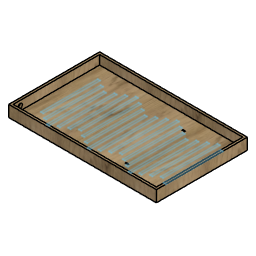
Dissertation_demo v1 v0 (Autodesk Fusion 360 design; units mm, degrees)
Autodesk Fusion 360 part; units mm, degrees
sketch "Sketch1" plane through (0, 0, 0) normal (0, 0, 1) x (1, 0, 0) in component "Component'"
  line L0 (211.4953, 133.158) -> (206.4953, 133.158)
  line L1 (206.4953, 133.158) -> (206.4953, 127.158)
  line L2 (206.4953, 127.158) -> (211.4953, 127.158)
  line L3 (211.4953, 127.158) -> (211.4953, 133.158)
  dimension "d10" = 5
  dimension "d11" = 6
  constraint horizontal L0
  constraint vertical L1
  constraint horizontal L2
  constraint vertical L3
  measures "d10" distance of L0.start L0.end
  measures "d11" distance of L0.start L2.end
extrude "Extrude1" add sketch "Sketch1" against normal blind 3 makes body 1 in component "Component'"
copy_body "CopyPasteBodies1" bodies 1 makes body 2 in component "Component'"
move_body "Move1" bodies 2 to x (1, 0, 0) y (0, 1, 0) z (0, 0, 1) at (0, -17, 0) in component "Component'"
copy_body "CopyPasteBodies2" bodies 1 2 makes body 3 makes body 4 in component "Component'"
move_body "Move2" bodies 3 4 to x (1, 0, 0) y (0, 1, 0) z (0, 0, 1) at (0, -35, 0) in component "Component'"
copy_body "CopyPasteBodies3" bodies 1 2 3 4 makes body 5 makes body 6 makes body 7 makes body 8 in component "Component'"
move_body "Move3" bodies 5 6 7 8 to x (1, 0, 0) y (0, 1, 0) z (0, 0, 1) at (0, -68, 0) in component "Component'"
copy_body "CopyPasteBodies4" bodies 1 2 3 4 5 6 7 makes body 9 makes body 10 makes body 11 makes body 12 makes body 13 makes body 14 makes body 15 in component "Component'"
move_body "Move4" bodies 9 10 11 12 13 14 15 to x (1, 0, 0) y (0, 1, 0) z (0, 0, 1) at (0, -136, 0) in component "Component'"
sketch "Sketch2" plane through (0, 0, 0) normal (0, 0, 1) x (1, 0, 0) in component "Component'"
  line L0 (213.9024, 135.458) -> (203.9024, 135.458)
  line L1 (203.9024, 135.458) -> (203.9024, -114.542)
  line L2 (203.9024, -114.542) -> (213.9024, -114.542)
  line L3 (213.9024, -114.542) -> (213.9024, 135.458)
  dimension "d14" = 10
  dimension "d15" = 250
  constraint horizontal L0
  constraint vertical L1
  constraint horizontal L2
  constraint vertical L3
  measures "d14" distance of L0.start L0.end
  measures "d15" distance of L0.start L2.end
extrude "Extrude2" cut sketch "Sketch2" against normal blind 1 bodies 1 2 3 4 5 6 7 8 9 10 11 12 13 14 15 in component "Component'"
move_body "Move5" bodies 1 2 3 4 5 6 7 9 8 10 12 13 14 15 11 to x (1, 0, 0) y (0, 1, 0) z (0, 0, 1) at (0, 0, -1) in component "Component'"
extrude "Extrude4" add sketch "Sketch2" against normal blind 1 separate body makes body 16 in component "Component'"
sketch "Sketch1 (2)" plane through (0, 0, 0) normal (0, 0, 1) x (1, 0, 0) in component "Main"
  line L0 (-250, 200) -> (250, 200)
  line L1 (250, 200) -> (250, -200)
  line L2 (250, -200) -> (-250, -200)
  line L3 (-250, -200) -> (-250, 200)
  line L4 (-250, 200) -> (250, -200) construction
  line L5 (250, 200) -> (-250, -200) construction
  line L6 (-240, 190) -> (240, 190)
  line L7 (240, 190) -> (240, -190)
  line L8 (240, -190) -> (-240, -190)
  line L9 (-240, -190) -> (-240, 190)
  dimension "d26" = 500
  dimension "d27" = 400
  dimension "d28" = 10
  constraint horizontal L0
  constraint perpendicular L0 L1
  constraint parallel L0 L2
  constraint parallel L1 L3
  constraint coincident L4 origin
  constraint coincident L5 origin
  measures "d26" distance of L1.end L2.end
  measures "d27" distance of L0.end L1.end
extrude "Extrude1'" add sketch "Sketch1 (2)" along normal blind 50 separate body makes body 17 in component "Main"
extrude "Extrude3" add sketch "Sketch1 (2)" along normal blind 10 contours L6 L7 L8 L9 bodies 17 in component "Main"
sketch "Sketch2 (2)" plane through (0, 0, 0) normal (0, 0, 1) x (1, 0, 0) in component "Main"
sketch "Sketch3" plane through (0, 0, 0) normal (0, 0, 1) x (1, 0, 0) in component "Main"
  line L0 (201, 127) -> (189, 127)
  line L1 (189, 127) -> (189, 123)
  line L2 (189, 123) -> (201, 123)
  line L3 (201, 123) -> (201, 127)
  dimension "d35" = 12
  dimension "d36" = 4
  constraint horizontal L0
  constraint vertical L1
  constraint horizontal L2
  constraint vertical L3
  measures "d35" distance of L0.start L0.end
  measures "d36" distance of L0.start L2.end
extrude "Extrude4'" cut sketch "Sketch3" along normal blind 10 bodies 17 in component "Main"
sketch "Sketch4" plane through (-13.9, -10.5, 0) normal (0, 0, 1) x (1, 0, 0) in component "Main"
  line L0 (214.9, -116.5) -> (202.9, -116.5)
  line L1 (202.9, -116.5) -> (202.9, -112.5)
  line L2 (202.9, -112.5) -> (214.9, -112.5)
  line L3 (214.9, -112.5) -> (214.9, -116.5)
  dimension "d39" = 12
  dimension "d40" = 4
  constraint horizontal L0
  constraint vertical L1
  constraint horizontal L2
  constraint vertical L3
  measures "d39" distance of L0.start L0.end
  measures "d40" distance of L0.start L2.end
extrude "Extrude5" cut sketch "Sketch4" along normal blind 10 bodies 17 in component "Main"
sketch "Sketch1 (3)" plane through (0, 0, 0) normal (0, 0, 1) x (1, 0, 0) in component "Component''"
  line L0 (202.6, 125) -> (187.4, 125)
  line L1 (187.4, 125) -> (187.4, -125)
  line L2 (187.4, -125) -> (202.6, -125)
  line L3 (202.6, -125) -> (202.6, 125)
  dimension "d43" = 15.2
  dimension "d44" = 250
  constraint horizontal L0
  constraint vertical L1
  constraint horizontal L2
  constraint vertical L3
  measures "d43" distance of L0.start L0.end
  measures "d44" distance of L0.start L2.end
extrude "Extrude1''" add sketch "Sketch1 (3)" against normal blind 5 separate body makes body 18 in component "Component''"
sketch "Sketch2 (3)" plane through (0, -125, 0) normal (0, -1, 0) x (1, 0, 0) in component "Component''"
  line L0 (202.6, 0) -> (187.4, 0)
  line L1 (187.4, 0) -> (187.4, -5)
  line L2 (187.4, -5) -> (202.6, -5)
  line L3 (202.6, -5) -> (202.6, 0)
  line L4 (202, 0) -> (188, 0)
  line L5 (188, 0) -> (188, -4)
  line L6 (188, -4) -> (202, -4)
  line L7 (202, -4) -> (202, 0)
  constraint horizontal L4
  constraint vertical L5
  constraint horizontal L6
  constraint vertical L7
  constraint coincident L0 L4.start
extrude "Extrude2'" cut sketch "Sketch2 (3)" against normal blind 250 contours L0 L4 L5 L6 L7 bodies 18 in component "Component''"
hole "Hole1" at (-250, -159.5585, 28.611) direction (1, 0, 0) diameter 20 depth 110 tip angle 118 bodies 17 in component "Main"
move_face "OffsetFaces1" offset 150 1 faces at (250, 66.6667, 33.3333) on bodies 17 in component "Main"
sketch "Sketch1 (4)" plane through (0, 0, 50) normal (0, 0, 1) x (-1, 0, 0)
  line L0 (-240, 190) -> (240, 190)
  line L1 (240, 190) -> (240, -190)
  line L2 (240, -190) -> (-240, -190)
  line L3 (-240, -190) -> (-240, 190)
  line L4 (250, 200) -> (-400, 200)
  line L5 (-400, 200) -> (-400, -200)
  line L6 (-400, -200) -> (250, -200)
  line L7 (250, -200) -> (250, 200)
  line L8 (-240, 190) -> (-390, 190)
  line L9 (-390, 190) -> (-390, -190)
  line L10 (-390, -190) -> (-240, -190)
  line L11 (-240, -190) -> (-240, 190)
  constraint horizontal L8
  constraint vertical L9
  constraint horizontal L10
  constraint vertical L11
  constraint coincident L0.start L3.end
extrude "Extrude6" cut sketch "Sketch1 (4)" against normal blind 40 contours L3 L8 L9 L10 L11 bodies 17 in component "Main"
sketch "Sketch2 (4)" plane through (0, 0, 0) normal (0, 0, -1) x (1, 0, 0)
  line L0 (201, 127) -> (201, 123)
  line L1 (201, 123) -> (189, 123)
  line L2 (189, 123) -> (189, 127)
  line L3 (189, 127) -> (201, 127)
  line L4 (189, -123) -> (201, -123)
  line L5 (201, -123) -> (201, -127)
  line L6 (201, -127) -> (189, -127)
  line L7 (189, -127) -> (189, -123)
  line L8 (400, 200) -> (-250, 200)
  line L9 (-250, 200) -> (-250, -200)
  line L10 (-250, -200) -> (400, -200)
  line L11 (400, -200) -> (400, 200)
  line L12 (374.7896, 142.4931) -> (372.7896, 142.4931)
  line L13 (372.7896, 142.4931) -> (372.7896, 162.4931)
  line L14 (372.7896, 162.4931) -> (374.7896, 162.4931)
  line L15 (374.7896, 162.4931) -> (374.7896, 142.4931)
  line L16 (352.7896, 162.4931) -> (352.7896, 142.4931)
  line L17 (352.7896, 142.4931) -> (350.7896, 142.4931)
  line L18 (350.7896, 142.4931) -> (350.7896, 162.4931)
  line L19 (350.7896, 162.4931) -> (352.7896, 162.4931)
  dimension "d55" = 2
  dimension "d56" = 20
  dimension "d59" = -22
  dimension "d60" = 0
  constraint horizontal L12
  constraint vertical L13
  constraint horizontal L14
  constraint vertical L15
  measures "d55" distance of L12.start L12.end
  measures "d56" distance of L12.start L14.end
extrude "Extrude7" cut sketch "Sketch2 (4)" against normal blind 49 contours L12 L13 L14 L15 | L16 L17 L18 L19 bodies 17 in component "Main"
sketch "Sketch3 (2)" plane through (0, 0, 0) normal (0, 0, -1) x (1, 0, 0)
  line L0 (372.7896, 142.4931) -> (372.7896, 162.4931)
  line L1 (372.7896, 162.4931) -> (374.7896, 162.4931)
  line L2 (374.7896, 162.4931) -> (374.7896, 142.4931)
  line L3 (374.7896, 142.4931) -> (372.7896, 142.4931)
  line L4 (352.7896, 142.4931) -> (350.7896, 142.4931)
  line L5 (350.7896, 142.4931) -> (350.7896, 162.4931)
  line L6 (350.7896, 162.4931) -> (352.7896, 162.4931)
  line L7 (352.7896, 162.4931) -> (352.7896, 142.4931)
  line L8 (201, 127) -> (201, 123)
  line L9 (201, 123) -> (189, 123)
  line L10 (189, 123) -> (189, 127)
  line L11 (189, 127) -> (201, 127)
  line L12 (189, -123) -> (201, -123)
  line L13 (201, -123) -> (201, -127)
  line L14 (201, -127) -> (189, -127)
  line L15 (189, -127) -> (189, -123)
  line L16 (400, 200) -> (-250, 200)
  line L17 (-250, 200) -> (-250, -200)
  line L18 (-250, -200) -> (400, -200)
  line L19 (400, -200) -> (400, 200)
  line L20 (370.7864, 140.5007) -> (368.7864, 140.5007)
  line L21 (368.7864, 140.5007) -> (368.7864, 164.5007)
  line L22 (368.7864, 164.5007) -> (370.7864, 164.5007)
  line L23 (370.7864, 164.5007) -> (370.7864, 140.5007)
  line L24 (356.7864, 140.5007) -> (354.7864, 140.5007)
  line L25 (356.7864, 164.5007) -> (356.7864, 140.5007)
  line L26 (354.7864, 140.5007) -> (354.7864, 164.5007)
  line L27 (354.7864, 164.5007) -> (356.7864, 164.5007)
  dimension "d63" = 2
  dimension "d64" = 24
  dimension "d67" = -14
  dimension "d68" = 0
  constraint horizontal L20
  constraint vertical L21
  constraint horizontal L22
  constraint vertical L23
  measures "d63" distance of L20.start L20.end
  measures "d64" distance of L20.start L22.end
extrude "Extrude8" cut sketch "Sketch3 (2)" against normal blind 12 contours L20 L21 L22 L23 | L24 L25 L26 L27 bodies 17 in component "Main"
sketch "Sketch4 (2)" plane through (0, 0, 0) normal (0, 0, -1) x (1, 0, 0)
  line L0 (368.7864, 140.5007) -> (368.7864, 164.5007)
  line L1 (368.7864, 164.5007) -> (370.7864, 164.5007)
  line L2 (370.7864, 164.5007) -> (370.7864, 140.5007)
  line L3 (370.7864, 140.5007) -> (368.7864, 140.5007)
  line L4 (356.7864, 140.5007) -> (354.7864, 140.5007)
  line L5 (354.7864, 140.5007) -> (354.7864, 164.5007)
  line L6 (354.7864, 164.5007) -> (356.7864, 164.5007)
  line L7 (356.7864, 164.5007) -> (356.7864, 140.5007)
  line L8 (372.7896, 142.4931) -> (372.7896, 162.4931)
  line L9 (372.7896, 162.4931) -> (374.7896, 162.4931)
  line L10 (374.7896, 162.4931) -> (374.7896, 142.4931)
  line L11 (374.7896, 142.4931) -> (372.7896, 142.4931)
  line L12 (352.7896, 142.4931) -> (350.7896, 142.4931)
  line L13 (350.7896, 142.4931) -> (350.7896, 162.4931)
  line L14 (350.7896, 162.4931) -> (352.7896, 162.4931)
  line L15 (352.7896, 162.4931) -> (352.7896, 142.4931)
  line L16 (201, 127) -> (201, 123)
  line L17 (201, 123) -> (189, 123)
  line L18 (189, 123) -> (189, 127)
  line L19 (189, 127) -> (201, 127)
  line L20 (189, -123) -> (201, -123)
  line L21 (201, -123) -> (201, -127)
  line L22 (201, -127) -> (189, -127)
  line L23 (189, -127) -> (189, -123)
  line L24 (400, 200) -> (-250, 200)
  line L25 (-250, 200) -> (-250, -200)
  line L26 (-250, -200) -> (400, -200)
  line L27 (400, -200) -> (400, 200)
  line L28 (366.8, 138.5) -> (364.8, 138.5)
  line L29 (364.8, 138.5) -> (364.8, 166.5)
  line L30 (364.8, 166.5) -> (366.8, 166.5)
  line L31 (366.8, 166.5) -> (366.8, 138.5)
  line L32 (360.8, 166.5) -> (360.8, 138.5)
  line L33 (360.8, 138.5) -> (358.8, 138.5)
  line L34 (358.8, 138.5) -> (358.8, 166.5)
  line L35 (358.8, 166.5) -> (360.8, 166.5)
  dimension "d73" = 2
  dimension "d74" = 28
  dimension "d77" = -6
  dimension "d78" = 0
  constraint horizontal L28
  constraint vertical L29
  constraint horizontal L30
  constraint vertical L31
  measures "d73" distance of L28.start L28.end
  measures "d74" distance of L28.start L30.end
sketch "Sketch5" plane through (0, 0, 0) normal (0, 0, -1) x (1, 0, 0)
  line L0 (367.5861, 138.8564) -> (365.5861, 138.8564)
  line L1 (365.5861, 138.8564) -> (365.5861, 166.8564)
  line L2 (365.5861, 166.8564) -> (367.5861, 166.8564)
  line L3 (367.5861, 166.8564) -> (367.5861, 138.8564)
  dimension "d71" = 2
  dimension "d72" = 28
  constraint horizontal L0
  constraint vertical L1
  constraint horizontal L2
  constraint vertical L3
  measures "d71" distance of L0.start L0.end
  measures "d72" distance of L0.start L2.end
extrude "Extrude9" cut sketch "Sketch4 (2)" against normal blind 10 contours L28 L29 L30 L31 | L32 L33 L34 L35 bodies 17 in component "Main"
sketch "Sketch6" plane through (0, 0, 0) normal (0, 0, -1) x (1, 0, 0)
  line L0 (364.8, 138.5) -> (364.8, 166.5)
  line L1 (364.8, 166.5) -> (366.8, 166.5)
  line L2 (366.8, 166.5) -> (366.8, 138.5)
  line L3 (366.8, 138.5) -> (364.8, 138.5)
  line L4 (360.8, 138.5) -> (358.8, 138.5)
  line L5 (358.8, 138.5) -> (358.8, 166.5)
  line L6 (358.8, 166.5) -> (360.8, 166.5)
  line L7 (360.8, 166.5) -> (360.8, 138.5)
  line L8 (368.7864, 140.5007) -> (368.7864, 164.5007)
  line L9 (368.7864, 164.5007) -> (370.7864, 164.5007)
  line L10 (370.7864, 164.5007) -> (370.7864, 140.5007)
  line L11 (370.7864, 140.5007) -> (368.7864, 140.5007)
  line L12 (356.7864, 140.5007) -> (354.7864, 140.5007)
  line L13 (354.7864, 140.5007) -> (354.7864, 164.5007)
  line L14 (354.7864, 164.5007) -> (356.7864, 164.5007)
  line L15 (356.7864, 164.5007) -> (356.7864, 140.5007)
  line L16 (372.7896, 142.4931) -> (372.7896, 162.4931)
  line L17 (372.7896, 162.4931) -> (374.7896, 162.4931)
  line L18 (374.7896, 162.4931) -> (374.7896, 142.4931)
  line L19 (374.7896, 142.4931) -> (372.7896, 142.4931)
  line L20 (352.7896, 142.4931) -> (350.7896, 142.4931)
  line L21 (350.7896, 142.4931) -> (350.7896, 162.4931)
  line L22 (350.7896, 162.4931) -> (352.7896, 162.4931)
  line L23 (352.7896, 162.4931) -> (352.7896, 142.4931)
  line L24 (201, 127) -> (201, 123)
  line L25 (201, 123) -> (189, 123)
  line L26 (189, 123) -> (189, 127)
  line L27 (189, 127) -> (201, 127)
  line L28 (189, -123) -> (201, -123)
  line L29 (201, -123) -> (201, -127)
  line L30 (201, -127) -> (189, -127)
  line L31 (189, -127) -> (189, -123)
  line L32 (400, 200) -> (-250, 200)
  line L33 (-250, 200) -> (-250, -200)
  line L34 (-250, -200) -> (400, -200)
  line L35 (400, -200) -> (400, 200)
  line L36 (363.7997, 136.5) -> (361.7997, 136.5)
  line L37 (361.7997, 136.5) -> (361.7997, 168.5)
  line L38 (361.7997, 168.5) -> (363.7997, 168.5)
  line L39 (363.7997, 168.5) -> (363.7997, 136.5)
  dimension "d81" = 2
  dimension "d82" = 32
  constraint horizontal L36
  constraint vertical L37
  constraint horizontal L38
  constraint vertical L39
  measures "d81" distance of L36.start L36.end
  measures "d82" distance of L36.start L38.end
extrude "Extrude10" cut sketch "Sketch6" against normal blind 31 contours L36 L37 L38 L39 bodies 17 in component "Main"
extrude "Extrude2''" [suppressed] in component "Main"
extrude "Extrude3'" [suppressed] in component "Component'"
sketch "Sketch1 (5)" plane through (0, 0, 0) normal (0, 0, -1) x (1, 0, 0) in component "Component"
  line L0 (140, 190) -> (-140, 190)
  line L1 (-140, 190) -> (-140, -190)
  line L2 (-140, -190) -> (140, -190)
  line L3 (140, -190) -> (140, 190)
  line L4 (120, -150) -> (110, -150)
  line L5 (110, -150) -> (110, 100)
  line L6 (110, 100) -> (120, 100)
  line L7 (120, 100) -> (120, -150)
  dimension "d8" = 10
  dimension "d9" = 250
  constraint horizontal L4
  constraint vertical L5
  constraint horizontal L6
  constraint vertical L7
  measures "d8" distance of L4.start L4.end
  measures "d9" distance of L4.start L6.end
component "Component'" placed x (1, 0, 0) y (0, 1, 0) z (0, 0, 1) at (-13.9, -10.5, 0)
component "Component'" placed x (1, 0, 0) y (0, 1, 0) z (0, 0, 1) at (-43.9, 6.5, 0)
component "Main" placed x (1, 0, 0) y (0, 1, 0) z (0, 0, 1) at (0, 0, 0)
component "Component'" placed x (1, 0, 0) y (0, 1, 0) z (0, 0, 1) at (-73.9, 23.5, 0)
component "Component'" placed x (1, 0, 0) y (0, 1, 0) z (0, 0, 1) at (-103.9, 6.5, 0)
component "Component'" placed x (1, 0, 0) y (0, 1, 0) z (0, 0, 1) at (-133.9, -10.5, 0)
component "Component'" placed x (1, 0, 0) y (0, 1, 0) z (0, 0, 1) at (-163.9, -27.5, 0)
component "Component'" placed x (1, 0, 0) y (0, 1, 0) z (0, 0, 1) at (-193.9, -10.5, 0)
component "Component'" placed x (1, 0, 0) y (0, 1, 0) z (0, 0, 1) at (-223.9, 6.5, 0)
component "Component'" placed x (1, 0, 0) y (0, 1, 0) z (0, 0, 1) at (-253.9, 23.5, 0)
component "Component'" placed x (1, 0, 0) y (0, 1, 0) z (0, 0, 1) at (-283.9, 6.5, 0)
component "Component'" placed x (1, 0, 0) y (0, 1, 0) z (0, 0, 1) at (-313.9, -10.5, 0)
component "Component'" placed x (1, 0, 0) y (0, 1, 0) z (0, 0, 1) at (-343.9, -27.5, 0)
component "Component'" placed x (1, 0, 0) y (0, 1, 0) z (0, 0, 1) at (-373.9, -10.5, 0)
component "Component'" placed x (1, 0, 0) y (0, 1, 0) z (0, 0, 1) at (-403.9, 6.5, 0)
component "Component'" placed x (1, 0, 0) y (0, 1, 0) z (0, 0, 1) at (16.1, -27.5, 0)
component "Component'" placed x (1, 0, 0) y (0, 1, 0) z (0, 0, 1) at (46.1, -10.5, 0)
component "Component'" placed x (1, 0, 0) y (0, 1, 0) z (0, 0, 1) at (76.1, 6.5, 0)
component "Component'" placed x (1, 0, 0) y (0, 1, 0) z (0, 0, 1) at (106.1, 23.5, 0)
component "Component'" placed x (1, 0, 0) y (0, 1, 0) z (0, 0, 1) at (136.1, 6.5, 0)
component "Component''" placed x (1, 0, 0) y (0, 1, 0) z (0, 0, 1) at (13.9, 10.5, 0) in component "Component'"
